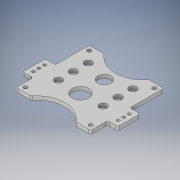
# Autodesk Inventor part: 2nd Plate
Saved by Autodesk Inventor 2018 (Build 220112000, 112)
## iProperties
Created: 2018-01-18
Part Number: 2nd Plate
Material: Generic
Document SubType Name: Modeling
Designer: maste
Density: 1 g/cm^3
Appearance: Default
Author: maste
Autodesk Inventor part; units mm, degrees
ref_plane "YZ Plane" through (0, 0, 0) normal (1, 0, 0) x (0, 1, 0)
ref_plane "XZ Plane" through (0, 0, 0) normal (0, 1, 0) x (-1, 0, 0)
ref_plane "XY Plane" through (0, 0, 0) normal (0, 0, 1) x (1, 0, 0)
sketch "Sketch1" plane through (0, 0, 0) normal (0, 1, 0) x (-1, 0, 0)
  line L0 (0, 0) -> (-127, 0)
  line L1 (-127, 0) -> (-127, -124.46)
  line L2 (-127, -124.46) -> (0, -124.46)
  line L3 (0, -124.46) -> (0, 0)
  dimension "d0" = 127
  dimension "d1" = 124.46
  constraints: 8 end point, 2 parallel, 1 horizontal, 1 perpendicular
  measures "d0" distance of L2.end L1.end
  measures "d1" distance of L0.end L1.end
extrude "Extrusion1" add sketch "Sketch1" along normal blind 6.35
sketch "Sketch2" plane through (0, 6.35, 0) normal (0, 1, 0) x (1, 0, 0)
  line L0 (127, 124.46) -> (0, 124.46) projected
  line L1 (0, 124.46) -> (7.9248, 124.46)
  line L2 (7.9248, 124.46) -> (7.9248, 116.5352)
  line L3 (0, 0) -> (127, 0) projected
  line L4 (127, 0) -> (119.0752, 0)
  line L5 (119.0752, 0) -> (119.0752, 7.9248)
  line L6 (0, 0) -> (7.9248, 0)
  line L7 (7.9248, 0) -> (7.9248, 7.9248)
  line L8 (127, 124.46) -> (119.0752, 124.46)
  line L9 (119.0752, 124.46) -> (119.0752, 116.5352)
  circle A0 centre (7.9248, 116.5352) radius 3.2512
  circle A1 centre (119.0752, 7.9248) radius 3.2512
  circle A2 centre (119.0752, 116.5352) radius 3.2512
  circle A3 centre (7.9248, 7.9248) radius 3.2512
  line L10 (0, 124.46) -> (25.4, 124.46)
  line L11 (25.4, 124.46) -> (25.4, 97.3582)
  line L12 (127, 0) -> (101.6, 0)
  line L13 (0, 0) -> (25.4, 0)
  line L14 (127, 124.46) -> (101.6, 124.46)
  line L15 (101.6, 124.46) -> (101.6, 97.3582)
  circle A4 centre (25.4, 97.3582) radius 6.35
  circle A5 centre (25.4, 46.5582) radius 6.35
  circle A6 centre (101.6, 46.5582) radius 6.35
  circle A7 centre (101.6, 97.3582) radius 6.35
  line L16 (25.4, 97.3582) -> (25.4, 71.9582)
  circle A8 centre (25.4, 71.9582) radius 6.35
  circle A9 centre (101.6, 71.9582) radius 6.35
  line L17 (0, 0) -> (63.5, 0)
  circle A10 centre (63.5, 46.0502) radius 14.2875
  line L18 (63.5, 46.0502) -> (63.5, 86.741)
  circle A11 centre (63.5, 86.741) radius 11.1125
  line L19 (127, 0) -> (127, 124.46) projected
  dimension "d4" = 7.9248
  dimension "d5" = 7.9248
  dimension "d6" = 7.9248
  dimension "d7" = 7.9248
  dimension "d8" = 6.5024
  dimension "d9" = 6.5024
  dimension "d10" = 25.4
  dimension "d11" = 27.1018
  dimension "d12" = 25.4
  dimension "d14" = 12.7
  dimension "d15" = 25.4
  dimension "d17" = 28.575
  dimension "d18" = 40.6908
  dimension "d66" = 27.1018
  dimension "d75" = 25.4
  dimension "d76" = 37.719
  dimension "d77" = 38.1
  dimension "d78" = 38.1
  dimension "d80" = 25.4
  dimension "d81" = 25.4
  dimension "d84" = 25.4
  constraints: 34 end point, 12 centre point, 8 coincident, 8 point on line, 5 vertical, 3 perpendicular, 1 midpoint
  measures "d4" distance of L0.end L1.end
  measures "d5" distance of L1.end L2.end
  measures "d6" distance of L3.end L4.end
  measures "d7" distance of L4.end L5.end
  measures "d8" diameter of A0
  measures "d9" diameter of A1
  measures "d10" distance of L0.end L10.end
  measures "d11" distance of L10.end L11.end
  measures "d12" distance of L3.end L12.end
  measures "d14" diameter of A4
  measures "d15" distance of L16.start L16.end
  measures "d17" diameter of A10
  measures "d18" distance of L18.start L18.end
  measures "d66" distance of L14.end L15.end
  measures "d75" distance of L15.end A9.centre
  measures "d76" distance from line of L0 L18.end
  measures "d77" horizontal distance of L18.start A6.centre
  measures "d78" horizontal distance of A5.centre L18.start
  measures "d80" distance of A5.centre L16.end
  measures "d81" distance of A6.centre A9.centre
  measures "d84" distance from line of L19 L15.end
extrude "Extrusion2" cut sketch "Sketch2" against normal blind 6.35
fillet "Fillet1" radius 3.175 4 edges at (127, 3.175, 0) (127, 3.175, -124.46) (0, 3.175, 0) (0, 3.175, -124.46)
sketch "Sketch6" plane through (0, 6.35, 0) normal (0, 1, 0) x (1, 0, 0)
  circle A0 centre (7.9248, 7.9248) radius 3.2512 projected
  line L0 (7.9248, 7.9248) -> (7.9248, 28.2448)
  line L1 (7.9248, 28.2448) -> (-3.1578, 28.2448)
  line L2 (-3.1578, 28.2448) -> (0, 28.575)
  line L3 (0, 121.285) -> (0, 3.175) projected
  line L4 (0, 28.575) -> (0, 66.675)
  line L5 (0, 66.675) -> (-17.4752, 66.675)
  line L6 (-17.4752, 66.675) -> (-17.4752, 28.575)
  line L7 (-17.4752, 28.575) -> (0, 28.575)
  line L8 (127, 3.175) -> (127, 121.285) projected
  line L9 (127, 28.575) -> (144.4752, 28.575)
  line L10 (144.4752, 28.575) -> (144.4752, 66.675)
  line L11 (144.4752, 66.675) -> (127, 66.675)
  line L12 (127, 66.675) -> (127, 28.575)
  line L13 (127, 28.575) -> (127, 31.75)
  circle A1 centre (119.0752, 7.9248) radius 3.2512 projected
  circle A2 centre (119.0752, 7.9248) radius 3.2512
  line L14 (3.175, 0) -> (123.825, 0) projected
  point P0 (0, 0)
  point P1 (0, 3.175)
  dimension "d47" = 3.175
  dimension "d48" = 38.1
  dimension "d49" = 17.4752
  dimension "d50" = 17.4752
  dimension "d67" = 3.175
  dimension "d69" = 38.1
  dimension "d82" = 28.575
  dimension "d83" = 28.575
  constraints: 24 end point, 4 perpendicular, 2 horizontal, 2 parallel, 2 point on line, 1 centre point, 1 coincident, 1 vertical, 3 other
  measures "d47" distance of L1.end L2.end
  measures "d48" distance of L2.end L4.end
  measures "d49" distance of L4.end L5.end
  measures "d50" distance of L11.end L10.end
  measures "d67" distance of L9.start L13.end
  measures "d69" distance between parallel lines of L11 L9
  measures "d82" distance from line of L7 point (0, 0)
  measures "d83" distance between parallel lines of L14 L9
extrude "Extrusion6" add sketch "Sketch6" against normal blind 6.35 contours L7 L6 L5 L3 | L8 L11 L10 L9
sketch "Sketch7" plane through (0, 6.35, 0) normal (0, 1, 0) x (1, 0, 0)
  line L0 (-17.4752, 28.575) -> (-17.4752, 66.675) projected
  line L1 (-17.4752, 66.675) -> (-8.7376, 66.675)
  line L2 (-17.4752, 66.675) -> (0, 66.675) projected
  line L3 (-8.7376, 66.675) -> (-8.7376, 28.575)
  line L4 (-17.4752, 28.575) -> (0, 28.575) projected
  line L5 (-8.7376, 66.675) -> (-8.7376, 57.15)
  line L6 (-8.7376, 57.15) -> (-8.7376, 47.625)
  line L7 (-8.7376, 47.625) -> (-8.7376, 38.1)
  circle A0 centre (-8.7376, 47.625) radius 2.54
  circle A1 centre (-8.7376, 57.15) radius 2.54
  circle A2 centre (-8.7376, 38.1) radius 2.54
  line L8 (144.4752, 66.675) -> (144.4752, 28.575) projected
  line L9 (144.4752, 57.15) -> (135.7376, 57.15)
  line L10 (144.4752, 47.625) -> (135.7376, 47.625)
  line L11 (144.4752, 38.1) -> (135.7376, 38.1)
  circle A3 centre (135.7376, 38.1) radius 2.54
  circle A4 centre (135.7376, 47.625) radius 2.54
  circle A5 centre (135.7376, 57.15) radius 2.54
  line L12 (144.4752, 66.675) -> (127, 66.675) projected
  point P0 (0, 0)
  dimension "d53" = 9.525
  dimension "d54" = 9.525
  dimension "d55" = 5.08
  dimension "d56" = 8.7376
  dimension "d70" = 9.525
  dimension "d71" = 9.525
  dimension "d72" = 9.525
  constraints: 16 end point, 6 centre point, 6 coincident, 4 midpoint, 4 point on line, 3 horizontal
  measures "d53" distance of L1.end L5.end
  measures "d54" distance of L6.end L7.end
  measures "d55" diameter of A0
  measures "d56" distance of L9.start L9.end
  measures "d70" distance from line of L12 L9.end
  measures "d71" distance of L10.end L9.end
  measures "d72" distance of L11.end L10.end
extrude "Extrusion7" cut sketch "Sketch7" against normal blind 6.35 contours A2 L3 | L3 A2 | A1 L3 | L3 A1 | A0 L3 | L3 A0 | A3 | A4 | A5
fillet "Fillet3" radius 3.175 8 edges at (127, 3.175, -28.575) (144.4752, 3.175, -28.575) (144.4752, 3.175, -66.675) (-17.4752, 3.175, -28.575) (127, 3.175, -66.675) (0, 3.175, -28.575) (-17.4752, 3.175, -66.675) (0, 3.175, -66.675)
sketch "Sketch8" plane through (0, 6.35, 0) normal (0, 1, 0) x (1, 0, 0)
  line L0 (123.825, 124.46) -> (3.175, 124.46) projected
  line L1 (63.5, 124.46) -> (63.5, 105.41)
  line L2 (63.5, 105.41) -> (25.4, 105.41)
  line L3 (25.4, 105.41) -> (101.6, 105.41)
  line L4 (25.4, 105.41) -> (25.4, 124.46)
  line L5 (101.6, 105.41) -> (101.6, 124.46)
  arc A0 (25.4, 124.46) -> (101.6, 124.46) centre (63.5, 153.035) ccw
  line L6 (3.175, 0) -> (123.825, 0) projected
  line L7 (25.4, 0) -> (101.6, 0)
  line L8 (63.5, 0) -> (63.5, 19.05)
  arc A1 (101.6, 0) -> (25.4, 0) centre (63.5, -28.575) ccw
  point P0 (0, 0)
  dimension "d60" = 19.05
  dimension "d61" = 38.1
  dimension "d62" = 76.2
  dimension "d63" = 19.05
  constraints: 14 end point, 6 point on circle, 5 point on line, 2 centre point, 2 midpoint, 2 perpendicular, 2 vertical, 1 parallel
  measures "d60" distance of L1.start L1.end
  measures "d61" distance of L1.end L2.end
  measures "d62" distance of L2.end L3.end
  measures "d63" distance of L8.start L8.end
extrude "Extrusion8" cut sketch "Sketch8" against normal blind 6.35 contours A0 L1 L0 | L1 A0 L0 | A1 L8 L6 | L8 A1 L6
fillet "Fillet4" radius 3.175 4 edges at (25.4, 3.175, -124.46) (101.6, 3.175, -124.46) (25.4, 3.175, 0) (101.6, 3.175, 0)
body "Solid1"
